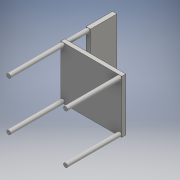
# Autodesk Inventor part: Chaise
Saved by Autodesk Inventor 2016 SP1 (Build 200210100, 210)
## iProperties
Created: 2016-10-04
Part Number: Chaise
Material: Générique
Document SubType Name: Modeling
Designer: dimercur
Density: 1 g/cm^3
Appearance: Par défaut
Author: dimercur
Autodesk Inventor part; units mm, degrees
ref_plane "YZ Plane" through (0, 0, 0) normal (1, 0, 0) x (0, 1, 0)
ref_plane "XZ Plane" through (0, 0, 0) normal (0, 1, 0) x (-1, 0, 0)
ref_plane "XY Plane" through (0, 0, 0) normal (0, 0, 1) x (1, 0, 0)
sketch "Esquisse1" plane through (0, 0, 0) normal (0, 1, 0) x (-1, 0, 0)
  line L0 (230, 200) -> (-230, 200)
  line L1 (-230, 200) -> (-230, -200)
  line L2 (-230, -200) -> (230, -200)
  line L3 (230, -200) -> (230, 200)
  point P0 (0, 0)
  dimension "d0" = 400
  dimension "d1" = 460
  dimension "d2" = 230
  dimension "d3" = 200
  constraints: 8 end point, 2 parallel, 1 horizontal, 1 perpendicular
  measures "d0" distance of L2.end L0.start
  measures "d1" distance of L0.start L0.end
  measures "d2" horizontal distance of point (0, 0) L0.start
  measures "d3" vertical distance of point (0, 0) L0.start
extrude "Extrusion1" add sketch "Esquisse1" along normal blind 30
sketch "Esquisse2" plane through (0, 0, 0) normal (0, -1, 0) x (1, 0, 0)
  circle A0 centre (215, 185) radius 15
  circle A1 centre (215, -185) radius 15
  circle A2 centre (-215, -185) radius 15
  circle A3 centre (-215, 185) radius 15
  line L0 (-230, 200) -> (230, 200) projected
  line L1 (230, 200) -> (230, -200) projected
  line L2 (230, -200) -> (-230, -200) projected
  line L3 (-230, -200) -> (-230, 200) projected
  point P0 (0, 0)
  dimension "d6" = 30
  dimension "d7" = 30
  dimension "d8" = 30
  dimension "d9" = 30
  dimension "d10" = 15
  dimension "d11" = 15
  dimension "d12" = 15
  dimension "d13" = 15
  dimension "d14" = 15
  dimension "d15" = 15
  dimension "d16" = 15
  dimension "d17" = 15
  constraints: 4 centre point
  measures "d6" diameter of A0
  measures "d7" diameter of A1
  measures "d8" diameter of A2
  measures "d9" diameter of A3
  measures "d10" distance from line of L0 A0.centre
  measures "d11" distance from line of L1 A0.centre
  measures "d12" distance from line of L1 A1.centre
  measures "d13" distance from line of L2 A1.centre
  measures "d14" distance from line of L3 A2.centre
  measures "d15" distance from line of L2 A2.centre
  measures "d16" distance from line of L3 A3.centre
  measures "d17" distance from line of A3.centre L0
extrude "Extrusion2" add sketch "Esquisse2" along normal blind 410 contours A0 | A1 | A3 | A2
sketch "Esquisse3" plane through (0, 30, 0) normal (0, 1, 0) x (1, 0, 0)
  arc A0 (-215, -200) -> (-230, -185) centre (-215, -185) ccw projected
  circle A1 centre (-215, -185) radius 15
  arc A2 (-230, 185) -> (-215, 200) centre (-215, 185) ccw projected
  circle A3 centre (-215, 185) radius 15
  point P0 (0, 0)
  constraints: 2 centre point, 2 coincident
extrude "Extrusion3" add sketch "Esquisse3" along normal blind 160
sketch "Esquisse4" plane through (-215, 190, 185) normal (0, 1, 0) x (1, 0, 0)
  line L0 (430, 385) -> (0, 385) projected
  line L1 (-15, -15) -> (18, -15)
  line L2 (18, -15) -> (18, 385)
  line L3 (18, 385) -> (-15, 385)
  line L4 (-15, 385) -> (-15, -15)
  point P0 (215, 185)
  dimension "d22" = 33
  constraints: 8 end point, 2 parallel, 1 horizontal, 1 perpendicular, 1 point on line
  measures "d22" distance between parallel lines of L2 L4
extrude "Extrusion4" add sketch "Esquisse4" along normal blind 200
equation "\"d2\" = 0.5 * d1"
equation "\"d3\" = 0.5 * d0"
equation "\"d7\" = d6"
equation "\"d8\" = d6"
equation "\"d9\" = d6"
equation "\"d12\" = d11"
equation "\"d13\" = d10"
equation "\"d14\" = d11"
equation "\"d15\" = d11"
equation "\"d16\" = d11"
equation "\"d17\" = d11"
